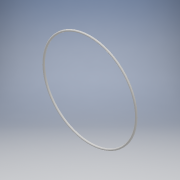
# Autodesk Inventor part: ConnectingRing
Saved by Autodesk Inventor 2018 (Build 220112000, 112)
## iProperties
Created: 2019-05-31
Part Number: ConnectingRing
Material: Generic
Document SubType Name: Modeling
Designer: ch1180245
Density: 1 g/cm^3
Appearance: Default
Author: ch1180245
Autodesk Inventor part; units mm, degrees
ref_plane "YZ Plane" through (0, 0, 0) normal (1, 0, 0) x (0, 1, 0)
ref_plane "XZ Plane" through (0, 0, 0) normal (0, 1, 0) x (-1, 0, 0)
ref_plane "XY Plane" through (0, 0, 0) normal (0, 0, 1) x (1, 0, 0)
sketch "Sketch1" plane through (0, 0, 0) normal (1, 0, 0) x (0, 1, 0)
  circle A0 centre (0.0356, -50) radius 1
  line L0 (-1.3645, 0) -> (1.4356, 0) projected
  point P0 (0, 0)
  dimension "d1" = 2
  dimension "d2" = 50
  constraints: 1 centre point
  measures "d1" diameter of A0
  measures "d2" distance of A0.centre point (0, 0)
revolve "Revolution1" add sketch "Sketch1" angle 360 about axis through (0, -10, 0) along (0, 1, 0)
body "Solid1"
